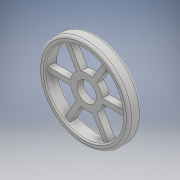
# Autodesk Inventor part: 앞바퀴2
Saved by Autodesk Inventor 2018 (Build 220112000, 112)
## iProperties
Created: 2019-11-13
Part Number: 앞바퀴2
Material: 일반
Document SubType Name: Modeling
Designer: LeeYounSeo
Density: 1 g/cm^3
Appearance: 기본값
Author: LeeYounSeo
Autodesk Inventor part; units mm, degrees
note: some values were not read from the file. Chosen so that the rebuilt part matches the saved one: arc direction of "돌출5".
ref_plane "YZ Plane" through (0, 0, 0) normal (1, 0, 0) x (0, 1, 0)
ref_plane "XZ Plane" through (0, 0, 0) normal (0, 1, 0) x (-1, 0, 0)
ref_plane "XY Plane" through (0, 0, 0) normal (0, 0, 1) x (1, 0, 0)
sketch "스케치1" plane through (0, 0, 0) normal (0, 1, 0) x (-1, 0, 0)
  circle A0 centre (0, 0) radius 37.5
  circle A1 centre (0, 0) radius 7.5
  circle A2 centre (0, 0) radius 12.5
  line L0 (2, 37.5) -> (-2, 37.5)
  line L1 (-2, 37.5) -> (-2, -37.5)
  line L2 (-2, -37.5) -> (2, -37.5)
  line L3 (2, -37.5) -> (2, 37.5)
  dimension "d0" = 75
  dimension "d1" = 15
  dimension "d2" = 25
  dimension "d3" = 2
  dimension "d4" = 2
  dimension "d5" = 75
  dimension "d6" = 37.5
  constraints: 8 end point, 3 centre point, 3 coincident, 2 parallel, 1 horizontal, 1 perpendicular
  measures "d0" diameter of A0
  measures "d1" diameter of A1
  measures "d2" diameter of A2
  measures "d3" distance from line of point (0, 0) L3
  measures "d4" distance from line of point (0, 0) L1
  measures "d5" distance between parallel lines of L2 L0
  measures "d6" distance from line of point (0, 0) L2
extrude "돌출1" add sketch "스케치1" along normal blind 5 contours L3 A1 L1 A2 | A2 L3 A1 | A2 L1 A1 L3 | L1 A1 A2
sketch "스케치2" plane through (0, 5, 0) normal (0, 1, 0) x (1, 0, 0)
  circle A0 centre (0, 0) radius 35
  circle A1 centre (0, 0) radius 30
  dimension "d9" = 70
  dimension "d10" = 60
  constraints: 2 centre point, 2 coincident
  measures "d9" diameter of A0
  measures "d10" diameter of A1
extrude "돌출2" add sketch "스케치2" against normal blind 7.5
sketch "스케치3" plane through (0, 5, 0) normal (0, 1, 0) x (1, 0, 0)
  circle A0 centre (0, 0) radius 30 projected
  circle A1 centre (0, 0) radius 35 projected
extrude "돌출3" add sketch "스케치3" along normal blind 2.5
sketch "스케치4" plane through (0, 5, 0) normal (0, 1, 0) x (1, 0, 0)
  line L0 (-34, -2) -> (34, -2)
  line L1 (34, -2) -> (34, 2)
  line L2 (34, 2) -> (-34, 2)
  line L3 (-34, 2) -> (-34, -2)
  point P0 (0, 0)
  dimension "d15" = 68
  dimension "d16" = 4
  dimension "d17" = 2
  dimension "d18" = 34
  constraints: 8 end point, 2 parallel, 1 horizontal, 1 perpendicular
  measures "d15" distance of L1.end L2.end
  measures "d16" distance of L0.end L1.end
  measures "d17" distance from line of point (0, 0) L2
  measures "d18" distance from line of point (0, 0) L1
extrude "돌출4" add sketch "스케치4" against normal blind 5
pattern_circular "원형 패턴1" count 6 over 360 about axis through (0, 0, 0) along (0, 1, 0) of "돌출4"
sketch "스케치5" plane through (0, 5, 0) normal (0, 1, 0) x (1, 0, 0)
  circle A0 centre (0, 0) radius 7.5
  arc A1 (1.8822, 7.26) -> (-1.8822, 7.26) centre (0, 0) ccw projected
  constraints: 1 centre point, 1 coincident
extrude "돌출5" cut sketch "스케치5" against normal blind 5
fillet "모깎기1" radius 2 2 edges at (-35, 7.5, 0) (-35, -2.5, 0)
fillet "모깎기2" radius 1 1 edges at (-30, 7.5, 0)
fillet "모깎기3" radius 1 1 edges at (-30, -2.5, 0)
